Autodesk Inventor part; units mm, degrees
(part 2 of 8)
  line L645 (-14.4464, -63.849) -> (-14.5331, -63.849) construction
  spline S62 degree 2 poles (-14.5331, -63.849) (-14.5782, -63.849) (-14.6233, -63.8281) knots 0 0 0 1 1 1
  line L646 (-14.5331, -63.849) -> (-14.5782, -63.849) construction
  line L647 (-14.5782, -63.849) -> (-14.6233, -63.8281) construction
  spline S63 degree 2 poles (-14.6233, -63.8281) (-14.8315, -63.7379) (-14.9598, -63.5714) knots 0 0 0 1 1 1
  line L648 (-14.6233, -63.8281) -> (-14.8315, -63.7379) construction
  line L649 (-14.8315, -63.7379) -> (-14.9598, -63.5714) construction
  spline S64 degree 2 poles (-14.9598, -63.5714) (-15.2096, -63.8455) (-15.5774, -63.8455) knots 0 0 0 1 1 1
  line L650 (-14.9598, -63.5714) -> (-15.2096, -63.8455) construction
  line L651 (-15.2096, -63.8455) -> (-15.5774, -63.8455) construction
  spline S65 degree 2 poles (-4.8151, -52.1801) (-5.2315, -52.1801) (-5.2315, -51.7638) knots 0 0 0 1 1 1
  line L652 (-4.8151, -52.1801) -> (-5.2315, -52.1801) construction
  line L653 (-5.2315, -52.1801) -> (-5.2315, -51.7638) construction
  spline S66 degree 2 poles (-5.2315, -51.7638) (-5.2315, -51.3475) (-4.8151, -51.3475) knots 0 0 0 1 1 1
  line L654 (-5.2315, -51.7638) -> (-5.2315, -51.3475) construction
  line L655 (-5.2315, -51.3475) -> (-4.8151, -51.3475) construction
  line L656 (-4.8151, -51.3475) -> (-1.4915, -51.3475)
  spline S67 degree 2 poles (-1.4915, -51.3475) (-1.0821, -51.3475) (-1.0821, -51.7638) knots 0 0 0 1 1 1
  line L657 (-1.4915, -51.3475) -> (-1.0821, -51.3475) construction
  line L658 (-1.0821, -51.3475) -> (-1.0821, -51.7638) construction
  spline S68 degree 2 poles (-1.0821, -51.7638) (-1.0821, -52.1801) (-1.4915, -52.1801) knots 0 0 0 1 1 1
  line L659 (-1.0821, -51.7638) -> (-1.0821, -52.1801) construction
  line L660 (-1.0821, -52.1801) -> (-1.4915, -52.1801) construction
  line L661 (-1.4915, -52.1801) -> (-4.8151, -52.1801)
  spline S69 degree 2 poles (-9.8734, -55.9243) (-10.0004, -55.9243) (-10.0766, -55.8058) knots 0 0 0 1 1 1
  line L662 (-9.8734, -55.9243) -> (-10.0004, -55.9243) construction
  line L663 (-10.0004, -55.9243) -> (-10.0766, -55.8058) construction
  spline S70 degree 2 poles (-11.6765, -55.8058) (-11.7527, -55.9243) (-11.8797, -55.9243) knots 0 0 0 1 1 1
  line L664 (-11.6765, -55.8058) -> (-11.7527, -55.9243) construction
  line L665 (-11.7527, -55.9243) -> (-11.8797, -55.9243) construction
  spline S71 degree 2 poles (-11.8797, -55.9243) (-11.9812, -55.9243) (-12.1463, -55.7719) (-12.1463, -55.6661) knots 0 0 0 1 2 2 2
  line L666 (-11.8797, -55.9243) -> (-11.9812, -55.9243) construction
  line L667 (-11.9812, -55.9243) -> (-12.1463, -55.7719) construction
  line L668 (-12.1463, -55.7719) -> (-12.1463, -55.6661) construction
  spline S72 degree 2 poles (-12.1463, -55.6661) (-12.1463, -55.5942) (-12.104, -55.5222) knots 0 0 0 1 1 1
  line L669 (-12.1463, -55.6661) -> (-12.1463, -55.5942) construction
  line L670 (-12.1463, -55.5942) -> (-12.104, -55.5222) construction
  spline S73 degree 2 poles (-12.104, -52.771) (-12.1463, -52.6991) (-12.1463, -52.6271) knots 0 0 0 1 1 1
  line L671 (-12.104, -52.771) -> (-12.1463, -52.6991) construction
  line L672 (-12.1463, -52.6991) -> (-12.1463, -52.6271) construction
  spline S74 degree 2 poles (-12.1463, -52.6271) (-12.1463, -52.5213) (-11.9812, -52.3689) (-11.8797, -52.3689) knots 0 0 0 1 2 2 2
  line L673 (-12.1463, -52.6271) -> (-12.1463, -52.5213) construction
  line L674 (-12.1463, -52.5213) -> (-11.9812, -52.3689) construction
  line L675 (-11.9812, -52.3689) -> (-11.8797, -52.3689) construction
  spline S75 degree 2 poles (-11.8797, -52.3689) (-11.7527, -52.3689) (-11.6765, -52.4875) knots 0 0 0 1 1 1
  line L676 (-11.8797, -52.3689) -> (-11.7527, -52.3689) construction
  line L677 (-11.7527, -52.3689) -> (-11.6765, -52.4875) construction
  spline S76 degree 2 poles (-10.0766, -52.4875) (-10.0004, -52.3689) (-9.8734, -52.3689) knots 0 0 0 1 1 1
  line L678 (-10.0766, -52.4875) -> (-10.0004, -52.3689) construction
  line L679 (-10.0004, -52.3689) -> (-9.8734, -52.3689) construction
  spline S77 degree 2 poles (-9.8734, -52.3689) (-9.7718, -52.3689) (-9.6025, -52.5213) (-9.6025, -52.6271) knots 0 0 0 1 2 2 2
  line L680 (-9.8734, -52.3689) -> (-9.7718, -52.3689) construction
  line L681 (-9.7718, -52.3689) -> (-9.6025, -52.5213) construction
  line L682 (-9.6025, -52.5213) -> (-9.6025, -52.6271) construction
  spline S78 degree 2 poles (-9.6025, -52.6271) (-9.6025, -52.6991) (-9.6491, -52.771) knots 0 0 0 1 1 1
  line L683 (-9.6025, -52.6271) -> (-9.6025, -52.6991) construction
  line L684 (-9.6025, -52.6991) -> (-9.6491, -52.771) construction
  spline S79 degree 2 poles (-9.6491, -55.5222) (-9.6025, -55.5942) (-9.6025, -55.6661) knots 0 0 0 1 1 1
  line L685 (-9.6491, -55.5222) -> (-9.6025, -55.5942) construction
  line L686 (-9.6025, -55.5942) -> (-9.6025, -55.6661) construction
  spline S80 degree 2 poles (-9.6025, -55.6661) (-9.6025, -55.7719) (-9.7718, -55.9243) (-9.8734, -55.9243) knots 0 0 0 1 2 2 2
  line L687 (-9.6025, -55.6661) -> (-9.6025, -55.7719) construction
  line L688 (-9.6025, -55.7719) -> (-9.7718, -55.9243) construction
  line L689 (-9.7718, -55.9243) -> (-9.8734, -55.9243) construction
  spline S81 degree 2 poles (-18.3701, -55.6314) (-18.4645, -55.9145) (-18.6809, -55.9145) knots 0 0 0 1 1 1
  line L690 (-18.3701, -55.6314) -> (-18.4645, -55.9145) construction
  line L691 (-18.4645, -55.9145) -> (-18.6809, -55.9145) construction
  spline S82 degree 2 poles (-18.6809, -55.9145) (-18.903, -55.9145) (-18.9918, -55.6314) knots 0 0 0 1 1 1
  line L692 (-18.6809, -55.9145) -> (-18.903, -55.9145) construction
  line L693 (-18.903, -55.9145) -> (-18.9918, -55.6314) construction
  line L694 (-18.9918, -55.6314) -> (-20.9901, -49.7141)
  spline S83 degree 2 poles (-20.9901, -49.7141) (-21.0068, -49.6531) (-21.0068, -49.592) knots 0 0 0 1 1 1
  line L695 (-20.9901, -49.7141) -> (-21.0068, -49.6531) construction
  line L696 (-21.0068, -49.6531) -> (-21.0068, -49.592) construction
  spline S84 degree 2 poles (-21.0068, -49.592) (-21.0068, -49.2756) (-20.6626, -49.2756) knots 0 0 0 1 1 1
  line L697 (-21.0068, -49.592) -> (-21.0068, -49.2756) construction
  line L698 (-21.0068, -49.2756) -> (-20.6626, -49.2756) construction
  spline S85 degree 2 poles (-20.6626, -49.2756) (-20.4406, -49.2756) (-20.3629, -49.5032) knots 0 0 0 1 1 1
  line L699 (-20.6626, -49.2756) -> (-20.4406, -49.2756) construction
  line L700 (-20.4406, -49.2756) -> (-20.3629, -49.5032) construction
  spline S86 degree 2 poles (-16.999, -49.5032) (-16.9213, -49.2756) (-16.6993, -49.2756) knots 0 0 0 1 1 1
  line L701 (-16.999, -49.5032) -> (-16.9213, -49.2756) construction
  line L702 (-16.9213, -49.2756) -> (-16.6993, -49.2756) construction
  spline S87 degree 2 poles (-16.6993, -49.2756) (-16.3551, -49.2756) (-16.3551, -49.592) knots 0 0 0 1 1 1
  line L703 (-16.6993, -49.2756) -> (-16.3551, -49.2756) construction
  line L704 (-16.3551, -49.2756) -> (-16.3551, -49.592) construction
  spline S88 degree 2 poles (-16.3551, -49.592) (-16.3551, -49.6531) (-16.3773, -49.7141) knots 0 0 0 1 1 1
  line L705 (-16.3551, -49.592) -> (-16.3551, -49.6531) construction
  line L706 (-16.3551, -49.6531) -> (-16.3773, -49.7141) construction
  line L707 (-16.3773, -49.7141) -> (-18.3701, -55.6314)
  spline S89 degree 2 poles (14.3835, -40.7072) (14.1892, -40.7072) (13.9706, -40.95) (13.9706, -41.12) knots 0 0 0 1 2 2 2
  line L708 (14.3835, -40.7072) -> (14.1892, -40.7072) construction
  line L709 (14.1892, -40.7072) -> (13.9706, -40.95) construction
  line L710 (13.9706, -40.95) -> (13.9706, -41.12) construction
  spline S90 degree 2 poles (13.9706, -41.12) (13.9706, -41.29) (14.0747, -41.408) knots 0 0 0 1 1 1
  line L711 (13.9706, -41.12) -> (13.9706, -41.29) construction
  line L712 (13.9706, -41.29) -> (14.0747, -41.408) construction
  spline S91 degree 2 poles (14.0747, -41.408) (14.1892, -41.5364) (14.3835, -41.5364) knots 0 0 0 1 1 1
  line L713 (14.0747, -41.408) -> (14.1892, -41.5364) construction
  line L714 (14.1892, -41.5364) -> (14.3835, -41.5364) construction
  spline S92 degree 2 poles (13.9359, -43.1045) (13.8735, -43.2016) (13.7694, -43.2016) knots 0 0 0 1 1 1
  line L715 (13.9359, -43.1045) -> (13.8735, -43.2016) construction
  line L716 (13.8735, -43.2016) -> (13.7694, -43.2016) construction
  spline S93 degree 2 poles (13.7694, -43.2016) (13.6826, -43.2016) (13.5508, -43.0767) (13.5508, -42.9935) knots 0 0 0 1 2 2 2
  line L717 (13.7694, -43.2016) -> (13.6826, -43.2016) construction
  line L718 (13.6826, -43.2016) -> (13.5508, -43.0767) construction
  line L719 (13.5508, -43.0767) -> (13.5508, -42.9935) construction
  spline S94 degree 2 poles (13.5508, -42.9935) (13.5508, -42.931) (13.589, -42.8755) knots 0 0 0 1 1 1
  line L720 (13.5508, -42.9935) -> (13.5508, -42.931) construction
  line L721 (13.5508, -42.931) -> (13.589, -42.8755) construction
  line L722 (13.589, -42.8755) -> (14.2135, -41.9388)
  spline S95 degree 2 poles (14.2135, -41.9388) (13.9012, -41.8868) (13.7173, -41.6404) knots 0 0 0 1 1 1
  line L723 (14.2135, -41.9388) -> (13.9012, -41.8868) construction
  line L724 (13.9012, -41.8868) -> (13.7173, -41.6404) construction
  spline S96 degree 2 poles (13.7173, -41.6404) (13.5543, -41.4184) (13.5543, -41.12) knots 0 0 0 1 1 1
  line L725 (13.7173, -41.6404) -> (13.5543, -41.4184) construction
  line L726 (13.5543, -41.4184) -> (13.5543, -41.12) construction
  spline S97 degree 2 poles (13.5543, -41.12) (13.5543, -40.7835) (13.7624, -40.5511) knots 0 0 0 1 1 1
  line L727 (13.5543, -41.12) -> (13.5543, -40.7835) construction
  line L728 (13.5543, -40.7835) -> (13.7624, -40.5511) construction
  spline S98 degree 2 poles (13.7624, -40.5511) (13.9914, -40.2909) (14.3835, -40.2909) knots 0 0 0 1 1 1
  line L729 (13.7624, -40.5511) -> (13.9914, -40.2909) construction
  line L730 (13.9914, -40.2909) -> (14.3835, -40.2909) construction
  line L731 (14.3835, -40.2909) -> (15.4208, -40.2909)
  spline S99 degree 2 poles (15.4208, -40.2909) (15.6289, -40.2909) (15.6289, -40.499) knots 0 0 0 1 1 1
  line L732 (15.4208, -40.2909) -> (15.6289, -40.2909) construction
  line L733 (15.6289, -40.2909) -> (15.6289, -40.499) construction
  line L734 (15.6289, -40.499) -> (15.6289, -42.99)
  spline S100 degree 2 poles (15.6289, -42.99) (15.6289, -43.1982) (15.4208, -43.1982) knots 0 0 0 1 1 1
  line L735 (15.6289, -42.99) -> (15.6289, -43.1982) construction
  line L736 (15.6289, -43.1982) -> (15.4208, -43.1982) construction
  spline S101 degree 2 poles (15.4208, -43.1982) (15.2126, -43.1982) (15.2126, -42.99) knots 0 0 0 1 1 1
  line L737 (15.4208, -43.1982) -> (15.2126, -43.1982) construction
  line L738 (15.2126, -43.1982) -> (15.2126, -42.99) construction
  spline S102 degree 2 poles (11.8925, -42.7819) (12.0625, -42.7819) (12.3053, -42.5355) (12.3053, -42.3655) knots 0 0 0 1 2 2 2
  line L739 (11.8925, -42.7819) -> (12.0625, -42.7819) construction
  line L740 (12.0625, -42.7819) -> (12.3053, -42.5355) construction
  line L741 (12.3053, -42.5355) -> (12.3053, -42.3655) construction
  spline S103 degree 2 poles (11.4762, -40.7072) (11.3062, -40.7072) (11.0633, -40.9535) (11.0633, -41.1235) knots 0 0 0 1 2 2 2
  line L742 (11.4762, -40.7072) -> (11.3062, -40.7072) construction
  line L743 (11.3062, -40.7072) -> (11.0633, -40.9535) construction
  line L744 (11.0633, -40.9535) -> (11.0633, -41.1235) construction
  line L745 (11.0633, -41.1235) -> (11.0633, -42.3655)
  spline S104 degree 2 poles (11.0633, -42.3655) (11.0633, -42.5355) (11.3062, -42.7819) (11.4762, -42.7819) knots 0 0 0 1 2 2 2
  line L746 (11.0633, -42.3655) -> (11.0633, -42.5355) construction
  line L747 (11.0633, -42.5355) -> (11.3062, -42.7819) construction
  line L748 (11.3062, -42.7819) -> (11.4762, -42.7819) construction
  line L749 (11.4762, -42.7819) -> (11.8925, -42.7819)
  line L750 (11.8925, -43.1982) -> (11.4762, -43.1982)
  spline S105 degree 2 poles (11.4762, -43.1982) (11.1362, -43.1982) (10.647, -42.7125) (10.647, -42.369) knots 0 0 0 1 2 2 2
  line L751 (11.4762, -43.1982) -> (11.1362, -43.1982) construction
  line L752 (11.1362, -43.1982) -> (10.647, -42.7125) construction
  line L753 (10.647, -42.7125) -> (10.647, -42.369) construction
  line L754 (10.647, -42.369) -> (10.647, -41.12)
  spline S106 degree 2 poles (10.647, -41.12) (10.647, -40.7766) (11.1362, -40.2909) (11.4762, -40.2909) knots 0 0 0 1 2 2 2
  line L755 (10.647, -41.12) -> (10.647, -40.7766) construction
  line L756 (10.647, -40.7766) -> (11.1362, -40.2909) construction
  line L757 (11.1362, -40.2909) -> (11.4762, -40.2909) construction
  line L758 (11.4762, -40.2909) -> (12.5135, -40.2909)
  spline S107 degree 2 poles (12.5135, -40.2909) (12.7216, -40.2909) (12.7216, -40.499) knots 0 0 0 1 1 1
  line L759 (12.5135, -40.2909) -> (12.7216, -40.2909) construction
  line L760 (12.7216, -40.2909) -> (12.7216, -40.499) construction
  line L761 (12.7216, -40.499) -> (12.7216, -42.3621)
  spline S108 degree 2 poles (12.7216, -42.3621) (12.7216, -42.6743) (13.0131, -42.7992) knots 0 0 0 1 1 1
  line L762 (12.7216, -42.3621) -> (12.7216, -42.6743) construction
  line L763 (12.7216, -42.6743) -> (13.0131, -42.7992) construction
  spline S109 degree 2 poles (13.0131, -42.7992) (13.1414, -42.8512) (13.1414, -42.9831) knots 0 0 0 1 1 1
  line L764 (13.0131, -42.7992) -> (13.1414, -42.8512) construction
  line L765 (13.1414, -42.8512) -> (13.1414, -42.9831) construction
  spline S110 degree 2 poles (13.1414, -42.9831) (13.1414, -43.0698) (13.0235, -43.2016) (12.9367, -43.2016) knots 0 0 0 1 2 2 2
  line L766 (13.1414, -42.9831) -> (13.1414, -43.0698) construction
  line L767 (13.1414, -43.0698) -> (13.0235, -43.2016) construction
  line L768 (13.0235, -43.2016) -> (12.9367, -43.2016) construction
  spline S111 degree 2 poles (12.9367, -43.2016) (12.8916, -43.2016) (12.8465, -43.1808) knots 0 0 0 1 1 1
  line L769 (12.9367, -43.2016) -> (12.8916, -43.2016) construction
  line L770 (12.8916, -43.2016) -> (12.8465, -43.1808) construction
  spline S112 degree 2 poles (12.8465, -43.1808) (12.6384, -43.0906) (12.51, -42.9241) knots 0 0 0 1 1 1
  line L771 (12.8465, -43.1808) -> (12.6384, -43.0906) construction
  line L772 (12.6384, -43.0906) -> (12.51, -42.9241) construction
  spline S113 degree 2 poles (12.51, -42.9241) (12.2602, -43.1982) (11.8925, -43.1982) knots 0 0 0 1 1 1
  line L773 (12.51, -42.9241) -> (12.2602, -43.1982) construction
  line L774 (12.2602, -43.1982) -> (11.8925, -43.1982) construction
  spline S114 degree 2 poles (-0.7775, -43.1982) (-0.9857, -43.1982) (-0.9857, -42.99) knots 0 0 0 1 1 1
  line L775 (-0.7775, -43.1982) -> (-0.9857, -43.1982) construction
  line L776 (-0.9857, -43.1982) -> (-0.9857, -42.99) construction
  spline S115 degree 2 poles (-2.2416, -43.0559) (-2.2867, -43.1982) (-2.4255, -43.1982) knots 0 0 0 1 1 1
  line L777 (-2.2416, -43.0559) -> (-2.2867, -43.1982) construction
  line L778 (-2.2867, -43.1982) -> (-2.4255, -43.1982) construction
  spline S116 degree 2 poles (-2.4255, -43.1982) (-2.644, -43.1982) (-2.644, -43.0004) knots 0 0 0 1 1 1
  line L779 (-2.4255, -43.1982) -> (-2.644, -43.1982) construction
  line L780 (-2.644, -43.1982) -> (-2.644, -43.0004) construction
  spline S117 degree 2 poles (-2.644, -43.0004) (-2.644, -42.9623) (-2.6301, -42.9241) knots 0 0 0 1 1 1
  line L781 (-2.644, -43.0004) -> (-2.644, -42.9623) construction
  line L782 (-2.644, -42.9623) -> (-2.6301, -42.9241) construction
  line L783 (-2.6301, -42.9241) -> (-1.8079, -40.4331)
  spline S118 degree 2 poles (-1.8079, -40.4331) (-1.7628, -40.2909) (-1.6136, -40.2909) knots 0 0 0 1 1 1
  line L784 (-1.8079, -40.4331) -> (-1.7628, -40.2909) construction
  line L785 (-1.7628, -40.2909) -> (-1.6136, -40.2909) construction
  line L786 (-1.6136, -40.2909) -> (-0.7775, -40.2909)
  spline S119 degree 2 poles (-0.7775, -40.2909) (-0.5694, -40.2909) (-0.5694, -40.499) knots 0 0 0 1 1 1
  line L787 (-0.7775, -40.2909) -> (-0.5694, -40.2909) construction
  line L788 (-0.5694, -40.2909) -> (-0.5694, -40.499) construction
  line L789 (-0.5694, -40.499) -> (-0.5694, -42.99)
  spline S120 degree 2 poles (-0.5694, -42.99) (-0.5694, -43.1982) (-0.7775, -43.1982) knots 0 0 0 1 1 1
  line L790 (-0.5694, -42.99) -> (-0.5694, -43.1982) construction
  line L791 (-0.5694, -43.1982) -> (-0.7775, -43.1982) construction
  spline S121 degree 2 poles (-12.4067, -43.1982) (-12.6149, -43.1982) (-12.6149, -42.99) knots 0 0 0 1 1 1
  line L792 (-12.4067, -43.1982) -> (-12.6149, -43.1982) construction
  line L793 (-12.6149, -43.1982) -> (-12.6149, -42.99) construction
  line L794 (-12.6149, -42.99) -> (-12.6149, -41.1235)
  spline S122 degree 2 poles (-12.6149, -41.1235) (-12.6149, -40.9535) (-12.8577, -40.7072) (-13.0277, -40.7072) knots 0 0 0 1 2 2 2
  line L795 (-12.6149, -41.1235) -> (-12.6149, -40.9535) construction
  line L796 (-12.6149, -40.9535) -> (-12.8577, -40.7072) construction
  line L797 (-12.8577, -40.7072) -> (-13.0277, -40.7072) construction
  spline S123 degree 2 poles (-13.8569, -42.99) (-13.8569, -43.1982) (-14.0651, -43.1982) knots 0 0 0 1 1 1
  line L798 (-13.8569, -42.99) -> (-13.8569, -43.1982) construction
  line L799 (-13.8569, -43.1982) -> (-14.0651, -43.1982) construction
  spline S124 degree 2 poles (-14.0651, -43.1982) (-14.2732, -43.1982) (-14.2732, -42.99) knots 0 0 0 1 1 1
  line L800 (-14.0651, -43.1982) -> (-14.2732, -43.1982) construction
  line L801 (-14.2732, -43.1982) -> (-14.2732, -42.99) construction
  line L802 (-14.2732, -42.99) -> (-14.2732, -40.499)
  spline S125 degree 2 poles (-14.2732, -40.499) (-14.2732, -40.2909) (-14.0651, -40.2909) knots 0 0 0 1 1 1
  line L803 (-14.2732, -40.499) -> (-14.2732, -40.2909) construction
  line L804 (-14.2732, -40.2909) -> (-14.0651, -40.2909) construction
  line L805 (-14.0651, -40.2909) -> (-13.0277, -40.2909)
  spline S126 degree 2 poles (-13.0277, -40.2909) (-12.6843, -40.2909) (-12.1986, -40.7766) (-12.1986, -41.12) knots 0 0 0 1 2 2 2
  line L806 (-13.0277, -40.2909) -> (-12.6843, -40.2909) construction
  line L807 (-12.6843, -40.2909) -> (-12.1986, -40.7766) construction
  line L808 (-12.1986, -40.7766) -> (-12.1986, -41.12) construction
  line L809 (-12.1986, -41.12) -> (-12.1986, -42.99)
  spline S127 degree 2 poles (-12.1986, -42.99) (-12.1986, -43.1982) (-12.4067, -43.1982) knots 0 0 0 1 1 1
  line L810 (-12.1986, -42.99) -> (-12.1986, -43.1982) construction
  line L811 (-12.1986, -43.1982) -> (-12.4067, -43.1982) construction
  spline S128 degree 2 poles (-15.935, -42.7819) (-15.765, -42.7819) (-15.5222, -42.5355) (-15.5222, -42.3655) knots 0 0 0 1 2 2 2
  line L812 (-15.935, -42.7819) -> (-15.765, -42.7819) construction
  line L813 (-15.765, -42.7819) -> (-15.5222, -42.5355) construction
  line L814 (-15.5222, -42.5355) -> (-15.5222, -42.3655) construction
  spline S129 degree 2 poles (-16.3514, -40.7072) (-16.5213, -40.7072) (-16.7642, -40.9535) (-16.7642, -41.1235) knots 0 0 0 1 2 2 2
  line L815 (-16.3514, -40.7072) -> (-16.5213, -40.7072) construction
  line L816 (-16.5213, -40.7072) -> (-16.7642, -40.9535) construction
  line L817 (-16.7642, -40.9535) -> (-16.7642, -41.1235) construction
  line L818 (-16.7642, -41.1235) -> (-16.7642, -42.3655)
  spline S130 degree 2 poles (-16.7642, -42.3655) (-16.7642, -42.5355) (-16.5213, -42.7819) (-16.3514, -42.7819) knots 0 0 0 1 2 2 2
  line L819 (-16.7642, -42.3655) -> (-16.7642, -42.5355) construction
  line L820 (-16.7642, -42.5355) -> (-16.5213, -42.7819) construction
  line L821 (-16.5213, -42.7819) -> (-16.3514, -42.7819) construction
  line L822 (-16.3514, -42.7819) -> (-15.935, -42.7819)
  line L823 (-15.935, -43.1982) -> (-16.3514, -43.1982)
  spline S131 degree 2 poles (-16.3514, -43.1982) (-16.6913, -43.1982) (-17.1805, -42.7125) (-17.1805, -42.369) knots 0 0 0 1 2 2 2
  line L824 (-16.3514, -43.1982) -> (-16.6913, -43.1982) construction
  line L825 (-16.6913, -43.1982) -> (-17.1805, -42.7125) construction
  line L826 (-17.1805, -42.7125) -> (-17.1805, -42.369) construction
  line L827 (-17.1805, -42.369) -> (-17.1805, -41.12)
  spline S132 degree 2 poles (-17.1805, -41.12) (-17.1805, -40.7766) (-16.6913, -40.2909) (-16.3514, -40.2909) knots 0 0 0 1 2 2 2
  line L828 (-17.1805, -41.12) -> (-17.1805, -40.7766) construction
  line L829 (-17.1805, -40.7766) -> (-16.6913, -40.2909) construction
  line L830 (-16.6913, -40.2909) -> (-16.3514, -40.2909) construction
  line L831 (-16.3514, -40.2909) -> (-15.314, -40.2909)
  spline S133 degree 2 poles (-15.314, -40.2909) (-15.1059, -40.2909) (-15.1059, -40.499) knots 0 0 0 1 1 1
  line L832 (-15.314, -40.2909) -> (-15.1059, -40.2909) construction
  line L833 (-15.1059, -40.2909) -> (-15.1059, -40.499) construction
  line L834 (-15.1059, -40.499) -> (-15.1059, -42.3621)
  spline S134 degree 2 poles (-15.1059, -42.3621) (-15.1059, -42.6743) (-14.8144, -42.7992) knots 0 0 0 1 1 1
  line L835 (-15.1059, -42.3621) -> (-15.1059, -42.6743) construction
  line L836 (-15.1059, -42.6743) -> (-14.8144, -42.7992) construction
  spline S135 degree 2 poles (-14.8144, -42.7992) (-14.6861, -42.8512) (-14.6861, -42.9831) knots 0 0 0 1 1 1
  line L837 (-14.8144, -42.7992) -> (-14.6861, -42.8512) construction
  line L838 (-14.6861, -42.8512) -> (-14.6861, -42.9831) construction
  spline S136 degree 2 poles (-14.6861, -42.9831) (-14.6861, -43.0698) (-14.804, -43.2016) (-14.8908, -43.2016) knots 0 0 0 1 2 2 2
  line L839 (-14.6861, -42.9831) -> (-14.6861, -43.0698) construction
  line L840 (-14.6861, -43.0698) -> (-14.804, -43.2016) construction
  line L841 (-14.804, -43.2016) -> (-14.8908, -43.2016) construction
  spline S137 degree 2 poles (-14.8908, -43.2016) (-14.9359, -43.2016) (-14.981, -43.1808) knots 0 0 0 1 1 1
  line L842 (-14.8908, -43.2016) -> (-14.9359, -43.2016) construction
  line L843 (-14.9359, -43.2016) -> (-14.981, -43.1808) construction
  spline S138 degree 2 poles (-14.981, -43.1808) (-15.1891, -43.0906) (-15.3175, -42.9241) knots 0 0 0 1 1 1
  line L844 (-14.981, -43.1808) -> (-15.1891, -43.0906) construction
  line L845 (-15.1891, -43.0906) -> (-15.3175, -42.9241) construction
  spline S139 degree 2 poles (-15.3175, -42.9241) (-15.5673, -43.1982) (-15.935, -43.1982) knots 0 0 0 1 1 1
  line L846 (-15.3175, -42.9241) -> (-15.5673, -43.1982) construction
  line L847 (-15.5673, -43.1982) -> (-15.935, -43.1982) construction
  spline S140 degree 2 poles (12.063, -33.4278) (11.723, -33.4278) (11.2304, -32.9421) (11.2304, -32.5987) knots 0 0 0 1 2 2 2
  line L848 (12.063, -33.4278) -> (11.723, -33.4278) construction
  line L849 (11.723, -33.4278) -> (11.2304, -32.9421) construction
  line L850 (11.2304, -32.9421) -> (11.2304, -32.5987) construction
  line L851 (11.2304, -32.5987) -> (11.2304, -31.3497)
  spline S141 degree 2 poles (11.2304, -31.3497) (11.2304, -31.0062) (11.723, -30.5205) (12.063, -30.5205) knots 0 0 0 1 2 2 2
  line L852 (11.2304, -31.3497) -> (11.2304, -31.0062) construction
  line L853 (11.2304, -31.0062) -> (11.723, -30.5205) construction
  line L854 (11.723, -30.5205) -> (12.063, -30.5205) construction
  line L855 (12.063, -30.5205) -> (12.684, -30.5205)
  spline S142 degree 2 poles (12.684, -30.5205) (12.8922, -30.5205) (12.8922, -30.7287) knots 0 0 0 1 1 1
  line L856 (12.684, -30.5205) -> (12.8922, -30.5205) construction
  line L857 (12.8922, -30.5205) -> (12.8922, -30.7287) construction
  spline S143 degree 2 poles (12.8922, -30.7287) (12.8922, -30.9369) (12.684, -30.9369) knots 0 0 0 1 1 1
  line L858 (12.8922, -30.7287) -> (12.8922, -30.9369) construction
  line L859 (12.8922, -30.9369) -> (12.684, -30.9369) construction
  line L860 (12.684, -30.9369) -> (12.063, -30.9369)
  spline S144 degree 2 poles (12.063, -30.9369) (11.893, -30.9369) (11.6467, -31.1832) (11.6467, -31.3532) knots 0 0 0 1 2 2 2
  line L861 (12.063, -30.9369) -> (11.893, -30.9369) construction
  line L862 (11.893, -30.9369) -> (11.6467, -31.1832) construction
  line L863 (11.6467, -31.1832) -> (11.6467, -31.3532) construction
  line L864 (11.6467, -31.3532) -> (11.6467, -32.5952)
  spline S145 degree 2 poles (11.6467, -32.5952) (11.6467, -32.7652) (11.893, -33.0115) (12.063, -33.0115) knots 0 0 0 1 2 2 2
  line L865 (11.6467, -32.5952) -> (11.6467, -32.7652) construction
  line L866 (11.6467, -32.7652) -> (11.893, -33.0115) construction
  line L867 (11.893, -33.0115) -> (12.063, -33.0115) construction
  line L868 (12.063, -33.0115) -> (12.684, -33.0115)
  spline S146 degree 2 poles (12.684, -33.0115) (12.8922, -33.0115) (12.8922, -33.2197) knots 0 0 0 1 1 1
  line L869 (12.684, -33.0115) -> (12.8922, -33.0115) construction
  line L870 (12.8922, -33.0115) -> (12.8922, -33.2197) construction
  spline S147 degree 2 poles (12.8922, -33.2197) (12.8922, -33.4278) (12.684, -33.4278) knots 0 0 0 1 1 1
  line L871 (12.8922, -33.2197) -> (12.8922, -33.4278) construction
  line L872 (12.8922, -33.4278) -> (12.684, -33.4278) construction
  line L873 (12.684, -33.4278) -> (12.063, -33.4278)
  spline S148 degree 2 poles (22.4086, -21.7323) (22.6167, -21.7323) (22.6167, -21.9405) knots 0 0 0 1 1 1
  line L874 (22.4086, -21.7323) -> (22.6167, -21.7323) construction
  line L875 (22.6167, -21.7323) -> (22.6167, -21.9405) construction
  spline S149 degree 2 poles (22.6167, -21.9405) (22.6167, -22.1486) (22.4086, -22.1486) knots 0 0 0 1 1 1
  line L876 (22.6167, -21.9405) -> (22.6167, -22.1486) construction
  line L877 (22.6167, -22.1486) -> (22.4086, -22.1486) construction
  spline S150 degree 2 poles (22.4086, -22.1486) (22.2004, -22.1486) (22.2004, -21.9405) knots 0 0 0 1 1 1
  line L878 (22.4086, -22.1486) -> (22.2004, -22.1486) construction
  line L879 (22.2004, -22.1486) -> (22.2004, -21.9405) construction
  spline S151 degree 2 poles (22.2004, -21.9405) (22.2004, -21.7323) (22.4086, -21.7323) knots 0 0 0 1 1 1
  line L880 (22.2004, -21.9405) -> (22.2004, -21.7323) construction
  line L881 (22.2004, -21.7323) -> (22.4086, -21.7323) construction
  spline S152 degree 2 poles (20.5386, -21.7323) (20.7086, -21.7323) (20.9515, -21.486) (20.9515, -21.316) knots 0 0 0 1 2 2 2
  line L882 (20.5386, -21.7323) -> (20.7086, -21.7323) construction
  line L883 (20.7086, -21.7323) -> (20.9515, -21.486) construction
  line L884 (20.9515, -21.486) -> (20.9515, -21.316) construction
  line L885 (20.9515, -21.316) -> (20.9515, -20.074)
  spline S153 degree 2 poles (20.9515, -20.074) (20.9515, -19.904) (20.7086, -19.6576) (20.5386, -19.6576) knots 0 0 0 1 2 2 2
  line L886 (20.9515, -20.074) -> (20.9515, -19.904) construction
  line L887 (20.9515, -19.904) -> (20.7086, -19.6576) construction
  line L888 (20.7086, -19.6576) -> (20.5386, -19.6576) construction
  spline S154 degree 2 poles (19.7094, -23.186) (19.7094, -23.3941) (19.5013, -23.3941) knots 0 0 0 1 1 1
  line L889 (19.7094, -23.186) -> (19.7094, -23.3941) construction
  line L890 (19.7094, -23.3941) -> (19.5013, -23.3941) construction
  spline S155 degree 2 poles (19.5013, -23.3941) (19.2931, -23.3941) (19.2931, -23.186) knots 0 0 0 1 1 1
  line L891 (19.5013, -23.3941) -> (19.2931, -23.3941) construction
  line L892 (19.2931, -23.3941) -> (19.2931, -23.186) construction
  line L893 (19.2931, -23.186) -> (19.2931, -19.4495)
  spline S156 degree 2 poles (19.2931, -19.4495) (19.2931, -19.2413) (19.5013, -19.2413) knots 0 0 0 1 1 1
  line L894 (19.2931, -19.4495) -> (19.2931, -19.2413) construction
  line L895 (19.2931, -19.2413) -> (19.5013, -19.2413) construction
  line L896 (19.5013, -19.2413) -> (20.5386, -19.2413)
  spline S157 degree 2 poles (20.5386, -19.2413) (20.8821, -19.2413) (21.3678, -19.727) (21.3678, -20.0705) knots 0 0 0 1 2 2 2
  line L897 (20.5386, -19.2413) -> (20.8821, -19.2413) construction
  line L898 (20.8821, -19.2413) -> (21.3678, -19.727) construction
  line L899 (21.3678, -19.727) -> (21.3678, -20.0705) construction
  line L900 (21.3678, -20.0705) -> (21.3678, -21.3195)
  spline S158 degree 2 poles (21.3678, -21.3195) (21.3678, -21.6629) (20.8821, -22.1486) (20.5386, -22.1486) knots 0 0 0 1 2 2 2
  line L901 (21.3678, -21.3195) -> (21.3678, -21.6629) construction
  line L902 (21.3678, -21.6629) -> (20.8821, -22.1486) construction
  line L903 (20.8821, -22.1486) -> (20.5386, -22.1486) construction
  spline S159 degree 2 poles (18.0442, -20.0705) (18.0442, -19.9005) (17.8013, -19.6576) (17.6313, -19.6576) knots 0 0 0 1 2 2 2
  line L904 (18.0442, -20.0705) -> (18.0442, -19.9005) construction
  line L905 (18.0442, -19.9005) -> (17.8013, -19.6576) construction
  line L906 (17.8013, -19.6576) -> (17.6313, -19.6576) construction
  line L907 (17.6313, -19.6576) -> (17.215, -19.6576)
  spline S160 degree 2 poles (17.215, -19.6576) (17.045, -19.6576) (16.8021, -19.9005) (16.8021, -20.0705) knots 0 0 0 1 2 2 2
  line L908 (17.215, -19.6576) -> (17.045, -19.6576) construction
  line L909 (17.045, -19.6576) -> (16.8021, -19.9005) construction
  line L910 (16.8021, -19.9005) -> (16.8021, -20.0705) construction
  spline S161 degree 2 poles (16.8021, -21.316) (16.8021, -21.486) (17.0485, -21.7323) (17.2185, -21.7323) knots 0 0 0 1 2 2 2
  line L911 (16.8021, -21.316) -> (16.8021, -21.486) construction
  line L912 (16.8021, -21.486) -> (17.0485, -21.7323) construction
  line L913 (17.0485, -21.7323) -> (17.2185, -21.7323) construction
  line L914 (17.2185, -21.7323) -> (18.2523, -21.7323)
  spline S162 degree 2 poles (18.2523, -21.7323) (18.4605, -21.7323) (18.4605, -21.9405) knots 0 0 0 1 1 1
  line L915 (18.2523, -21.7323) -> (18.4605, -21.7323) construction
  line L916 (18.4605, -21.7323) -> (18.4605, -21.9405) construction
  spline S163 degree 2 poles (18.4605, -21.9405) (18.4605, -22.1486) (18.2523, -22.1486) knots 0 0 0 1 1 1
  line L917 (18.4605, -21.9405) -> (18.4605, -22.1486) construction
  line L918 (18.4605, -22.1486) -> (18.2523, -22.1486) construction
  line L919 (18.2523, -22.1486) -> (17.215, -22.1486)
  spline S164 degree 2 poles (17.215, -22.1486) (16.8715, -22.1486) (16.3858, -21.6629) (16.3858, -21.3195) knots 0 0 0 1 2 2 2
  line L920 (17.215, -22.1486) -> (16.8715, -22.1486) construction
  line L921 (16.8715, -22.1486) -> (16.3858, -21.6629) construction
  line L922 (16.3858, -21.6629) -> (16.3858, -21.3195) construction
  line L923 (16.3858, -21.3195) -> (16.3858, -20.0705)
  spline S165 degree 2 poles (16.3858, -20.0705) (16.3858, -19.727) (16.8715, -19.2413) (17.215, -19.2413) knots 0 0 0 1 2 2 2
  line L924 (16.3858, -20.0705) -> (16.3858, -19.727) construction
  line L925 (16.3858, -19.727) -> (16.8715, -19.2413) construction
  line L926 (16.8715, -19.2413) -> (17.215, -19.2413) construction
  line L927 (17.215, -19.2413) -> (17.6313, -19.2413)
  spline S166 degree 2 poles (17.6313, -19.2413) (17.9748, -19.2413) (18.4605, -19.727) (18.4605, -20.0705) knots 0 0 0 1 2 2 2
  line L928 (17.6313, -19.2413) -> (17.9748, -19.2413) construction
  line L929 (17.9748, -19.2413) -> (18.4605, -19.727) construction
  line L930 (18.4605, -19.727) -> (18.4605, -20.0705) construction
  line L931 (18.4605, -20.0705) -> (18.4605, -20.695)
  spline S167 degree 2 poles (18.4605, -20.695) (18.4605, -20.9031) (18.2523, -20.9031) knots 0 0 0 1 1 1
  line L932 (18.4605, -20.695) -> (18.4605, -20.9031) construction
  line L933 (18.4605, -20.9031) -> (18.2523, -20.9031) construction
  spline S168 degree 2 poles (11.1922, -20.9031) (10.9841, -20.9031) (10.9841, -20.695) knots 0 0 0 1 1 1
  line L934 (11.1922, -20.9031) -> (10.9841, -20.9031) construction
  line L935 (10.9841, -20.9031) -> (10.9841, -20.695) construction
  spline S169 degree 2 poles (10.9841, -20.695) (10.9841, -20.4868) (11.1922, -20.4868) knots 0 0 0 1 1 1
  line L936 (10.9841, -20.695) -> (10.9841, -20.4868) construction
  line L937 (10.9841, -20.4868) -> (11.1922, -20.4868) construction
  line L938 (11.1922, -20.4868) -> (11.4004, -20.4868)
  spline S170 degree 2 poles (11.4004, -20.4868) (11.5947, -20.4868) (11.7092, -20.3585) knots 0 0 0 1 1 1
  line L939 (11.4004, -20.4868) -> (11.5947, -20.4868) construction
  line L940 (11.5947, -20.4868) -> (11.7092, -20.3585) construction
  spline S171 degree 2 poles (11.7092, -20.3585) (11.8132, -20.2405) (11.8132, -20.0705) knots 0 0 0 1 1 1
  line L941 (11.7092, -20.3585) -> (11.8132, -20.2405) construction
  line L942 (11.8132, -20.2405) -> (11.8132, -20.0705) construction
  spline S172 degree 2 poles (11.8132, -20.0705) (11.8132, -19.9005) (11.7092, -19.786) knots 0 0 0 1 1 1
  line L943 (11.8132, -20.0705) -> (11.8132, -19.9005) construction
  line L944 (11.8132, -19.9005) -> (11.7092, -19.786) construction
  spline S173 degree 2 poles (11.7092, -19.786) (11.5947, -19.6576) (11.3969, -19.6576) knots 0 0 0 1 1 1
  line L945 (11.7092, -19.786) -> (11.5947, -19.6576) construction
  line L946 (11.5947, -19.6576) -> (11.3969, -19.6576) construction
  line L947 (11.3969, -19.6576) -> (11.1888, -19.6576)
  spline S174 degree 2 poles (11.1888, -19.6576) (10.9078, -19.6576) (10.6927, -19.8242) knots 0 0 0 1 1 1
  line L948 (11.1888, -19.6576) -> (10.9078, -19.6576) construction
  line L949 (10.9078, -19.6576) -> (10.6927, -19.8242) construction
  spline S175 degree 2 poles (10.6927, -19.8242) (10.6302, -19.8693) (10.5643, -19.8693) knots 0 0 0 1 1 1
  line L950 (10.6927, -19.8242) -> (10.6302, -19.8693) construction
  line L951 (10.6302, -19.8693) -> (10.5643, -19.8693) construction
  spline S176 degree 2 poles (10.5643, -19.8693) (10.481, -19.8693) (10.3561, -19.7409) (10.3561, -19.6542) knots 0 0 0 1 2 2 2
  line L952 (10.5643, -19.8693) -> (10.481, -19.8693) construction
  line L953 (10.481, -19.8693) -> (10.3561, -19.7409) construction
  line L954 (10.3561, -19.7409) -> (10.3561, -19.6542) construction
  spline S177 degree 2 poles (10.3561, -19.6542) (10.3561, -19.557) (10.4429, -19.4911) knots 0 0 0 1 1 1
  line L955 (10.3561, -19.6542) -> (10.3561, -19.557) construction
  line L956 (10.3561, -19.557) -> (10.4429, -19.4911) construction
  spline S178 degree 2 poles (10.4429, -19.4911) (10.7655, -19.2413) (11.1888, -19.2413) knots 0 0 0 1 1 1
  line L957 (10.4429, -19.4911) -> (10.7655, -19.2413) construction
  line L958 (10.7655, -19.2413) -> (11.1888, -19.2413) construction
  line L959 (11.1888, -19.2413) -> (11.3969, -19.2413)
  spline S179 degree 2 poles (11.3969, -19.2413) (11.789, -19.2413) (12.0214, -19.4981) knots 0 0 0 1 1 1
  line L960 (11.3969, -19.2413) -> (11.789, -19.2413) construction
  line L961 (11.789, -19.2413) -> (12.0214, -19.4981) construction
  spline S180 degree 2 poles (12.0214, -19.4981) (12.2296, -19.734) (12.2296, -20.0705) knots 0 0 0 1 1 1
  line L962 (12.0214, -19.4981) -> (12.2296, -19.734) construction
  line L963 (12.2296, -19.734) -> (12.2296, -20.0705) construction
  spline S181 degree 2 poles (12.2296, -20.0705) (12.2296, -20.4556) (11.9694, -20.695) knots 0 0 0 1 1 1
  line L964 (12.2296, -20.0705) -> (12.2296, -20.4556) construction
  line L965 (12.2296, -20.4556) -> (11.9694, -20.695) construction
  spline S182 degree 2 poles (11.9694, -20.695) (12.2296, -20.9344) (12.2296, -21.3195) knots 0 0 0 1 1 1
  line L966 (11.9694, -20.695) -> (12.2296, -20.9344) construction
  line L967 (12.2296, -20.9344) -> (12.2296, -21.3195) construction
  spline S183 degree 2 poles (12.2296, -21.3195) (12.2296, -21.6594) (12.0214, -21.8919) knots 0 0 0 1 1 1
  line L968 (12.2296, -21.3195) -> (12.2296, -21.6594) construction
  line L969 (12.2296, -21.6594) -> (12.0214, -21.8919) construction
  spline S184 degree 2 poles (12.0214, -21.8919) (11.789, -22.1486) (11.3969, -22.1486) knots 0 0 0 1 1 1
  line L970 (12.0214, -21.8919) -> (11.789, -22.1486) construction
  line L971 (11.789, -22.1486) -> (11.3969, -22.1486) construction
  line L972 (11.3969, -22.1486) -> (11.1888, -22.1486)
  spline S185 degree 2 poles (11.1888, -22.1486) (10.7655, -22.1486) (10.4429, -21.8988) knots 0 0 0 1 1 1
  line L973 (11.1888, -22.1486) -> (10.7655, -22.1486) construction
  line L974 (10.7655, -22.1486) -> (10.4429, -21.8988) construction
  spline S186 degree 2 poles (10.4429, -21.8988) (10.3561, -21.8329) (10.3561, -21.7358) knots 0 0 0 1 1 1
  line L975 (10.4429, -21.8988) -> (10.3561, -21.8329) construction
  line L976 (10.3561, -21.8329) -> (10.3561, -21.7358) construction
  spline S187 degree 2 poles (10.3561, -21.7358) (10.3561, -21.649) (10.481, -21.5207) (10.5643, -21.5207) knots 0 0 0 1 2 2 2
  line L977 (10.3561, -21.7358) -> (10.3561, -21.649) construction
  line L978 (10.3561, -21.649) -> (10.481, -21.5207) construction
  line L979 (10.481, -21.5207) -> (10.5643, -21.5207) construction
  spline S188 degree 2 poles (10.5643, -21.5207) (10.6302, -21.5207) (10.6927, -21.5658) knots 0 0 0 1 1 1
  line L980 (10.5643, -21.5207) -> (10.6302, -21.5207) construction
  line L981 (10.6302, -21.5207) -> (10.6927, -21.5658) construction
  spline S189 degree 2 poles (10.6927, -21.5658) (10.9078, -21.7323) (11.1888, -21.7323) knots 0 0 0 1 1 1
  line L982 (10.6927, -21.5658) -> (10.9078, -21.7323) construction
  line L983 (10.9078, -21.7323) -> (11.1888, -21.7323) construction
  line L984 (11.1888, -21.7323) -> (11.3969, -21.7323)
  spline S190 degree 2 poles (11.3969, -21.7323) (11.5947, -21.7323) (11.7092, -21.6005) knots 0 0 0 1 1 1
  line L985 (11.3969, -21.7323) -> (11.5947, -21.7323) construction
  line L986 (11.5947, -21.7323) -> (11.7092, -21.6005) construction
  spline S191 degree 2 poles (11.7092, -21.6005) (11.8132, -21.4825) (11.8132, -21.3125) knots 0 0 0 1 1 1
  line L987 (11.7092, -21.6005) -> (11.8132, -21.4825) construction
  line L988 (11.8132, -21.4825) -> (11.8132, -21.3125) construction
  spline S192 degree 2 poles (11.8132, -21.3125) (11.8132, -20.9413) (11.4524, -20.9031) knots 0 0 0 1 1 1
  line L989 (11.8132, -21.3125) -> (11.8132, -20.9413) construction
  line L990 (11.8132, -20.9413) -> (11.4524, -20.9031) construction
  line L991 (11.4524, -20.9031) -> (11.1922, -20.9031)
  spline S193 degree 2 poles (-18.3883, -34.8092) (-18.5964, -34.8092) (-18.5964, -34.601) knots 0 0 0 1 1 1
  line L992 (-18.3883, -34.8092) -> (-18.5964, -34.8092) construction
  line L993 (-18.5964, -34.8092) -> (-18.5964, -34.601) construction
  line L994 (-18.5964, -34.601) -> (-18.5964, -30.8646)
  spline S194 degree 2 poles (-18.5964, -30.8646) (-18.5964, -30.6564) (-18.3883, -30.6564) knots 0 0 0 1 1 1
  line L995 (-18.5964, -30.8646) -> (-18.5964, -30.6564) construction
  line L996 (-18.5964, -30.6564) -> (-18.3883, -30.6564) construction
  spline S195 degree 2 poles (-18.3883, -30.6564) (-18.1801, -30.6564) (-18.1801, -30.8646) knots 0 0 0 1 1 1
  line L997 (-18.3883, -30.6564) -> (-18.1801, -30.6564) construction
  line L998 (-18.1801, -30.6564) -> (-18.1801, -30.8646) construction
  spline S196 degree 2 poles (-16.7265, -34.3929) (-16.5183, -34.3929) (-16.5183, -34.601) knots 0 0 0 1 1 1
  line L999 (-16.7265, -34.3929) -> (-16.5183, -34.3929) construction
  line L1000 (-16.5183, -34.3929) -> (-16.5183, -34.601) construction
  spline S197 degree 2 poles (-16.5183, -34.601) (-16.5183, -34.8092) (-16.7265, -34.8092) knots 0 0 0 1 1 1
  line L1001 (-16.5183, -34.601) -> (-16.5183, -34.8092) construction
  line L1002 (-16.5183, -34.8092) -> (-16.7265, -34.8092) construction
  line L1003 (-16.7265, -34.8092) -> (-18.3883, -34.8092)
  spline S198 degree 2 poles (-19.795, -25.6945) (-19.795, -25.7777) (-19.9199, -25.9096) (-20.0032, -25.9096) knots 0 0 0 1 2 2 2
  line L1004 (-19.795, -25.6945) -> (-19.795, -25.7777) construction
  line L1005 (-19.795, -25.7777) -> (-19.9199, -25.9096) construction
  line L1006 (-19.9199, -25.9096) -> (-20.0032, -25.9096) construction
  spline S199 degree 2 poles (-20.0032, -25.9096) (-20.0691, -25.9096) (-20.1281, -25.8679) knots 0 0 0 1 1 1
  line L1007 (-20.0032, -25.9096) -> (-20.0691, -25.9096) construction
  line L1008 (-20.0691, -25.9096) -> (-20.1281, -25.8679) construction
  spline S200 degree 2 poles (-20.1281, -25.8679) (-20.5236, -25.5834) (-21.0058, -25.5834) knots 0 0 0 1 1 1
  line L1009 (-20.1281, -25.8679) -> (-20.5236, -25.5834) construction
  line L1010 (-20.5236, -25.5834) -> (-21.0058, -25.5834) construction
  spline S201 degree 2 poles (-21.0058, -25.5834) (-21.3181, -25.5834) (-21.8211, -25.8436) (-21.8211, -26.0934) knots 0 0 0 1 2 2 2
  line L1011 (-21.0058, -25.5834) -> (-21.3181, -25.5834) construction
  line L1012 (-21.3181, -25.5834) -> (-21.8211, -25.8436) construction
  line L1013 (-21.8211, -25.8436) -> (-21.8211, -26.0934) construction
  spline S202 degree 2 poles (-21.8211, -26.0934) (-21.8211, -26.2426) (-21.7031, -26.3328) knots 0 0 0 1 1 1
  line L1014 (-21.8211, -26.0934) -> (-21.8211, -26.2426) construction
  line L1015 (-21.8211, -26.2426) -> (-21.7031, -26.3328) construction
  line L1016 (-21.7031, -26.3328) -> (-20.1628, -27.4708)
  spline S203 degree 2 poles (-20.1628, -27.4708) (-19.7464, -27.7761) (-19.7464, -28.3242) knots 0 0 0 1 1 1
  line L1017 (-20.1628, -27.4708) -> (-19.7464, -27.7761) construction
  line L1018 (-19.7464, -27.7761) -> (-19.7464, -28.3242) construction
  spline S204 degree 2 poles (-19.7464, -28.3242) (-19.7464, -28.8932) (-20.6207, -29.3511) (-21.0405, -29.3511) knots 0 0 0 1 2 2 2
  line L1019 (-19.7464, -28.3242) -> (-19.7464, -28.8932) construction
  line L1020 (-19.7464, -28.8932) -> (-20.6207, -29.3511) construction
  line L1021 (-20.6207, -29.3511) -> (-21.0405, -29.3511) construction
  spline S205 degree 2 poles (-21.0405, -29.3511) (-21.5678, -29.3511) (-22.1403, -28.9799) knots 0 0 0 1 1 1
  line L1022 (-21.0405, -29.3511) -> (-21.5678, -29.3511) construction
  line L1023 (-21.5678, -29.3511) -> (-22.1403, -28.9799) construction
  spline S206 degree 2 poles (-22.1403, -28.9799) (-22.2374, -28.9175) (-22.2374, -28.8134) knots 0 0 0 1 1 1
  line L1024 (-22.1403, -28.9799) -> (-22.2374, -28.9175) construction
  line L1025 (-22.2374, -28.9175) -> (-22.2374, -28.8134) construction
  spline S207 degree 2 poles (-22.2374, -28.8134) (-22.2374, -28.7267) (-22.116, -28.5948) (-22.0293, -28.5948) knots 0 0 0 1 2 2 2
  line L1026 (-22.2374, -28.8134) -> (-22.2374, -28.7267) construction
  line L1027 (-22.2374, -28.7267) -> (-22.116, -28.5948) construction
  line L1028 (-22.116, -28.5948) -> (-22.0293, -28.5948) construction
  spline S208 degree 2 poles (-22.0293, -28.5948) (-21.9703, -28.5948) (-21.9182, -28.633) knots 0 0 0 1 1 1
  line L1029 (-22.0293, -28.5948) -> (-21.9703, -28.5948) construction
  line L1030 (-21.9703, -28.5948) -> (-21.9182, -28.633) construction
  spline S209 degree 2 poles (-21.9182, -28.633) (-21.4464, -28.9348) (-21.0301, -28.9348) knots 0 0 0 1 1 1
  line L1031 (-21.9182, -28.633) -> (-21.4464, -28.9348) construction
  line L1032 (-21.4464, -28.9348) -> (-21.0301, -28.9348) construction
  spline S210 degree 2 poles (-21.0301, -28.9348) (-20.7109, -28.9348) (-20.3744, -28.7614) knots 0 0 0 1 1 1
  line L1033 (-21.0301, -28.9348) -> (-20.7109, -28.9348) construction
  line L1034 (-20.7109, -28.9348) -> (-20.3744, -28.7614) construction
  spline S211 degree 2 poles (-20.3744, -28.7614) (-20.1489, -28.6399) (-20.1489, -28.3312) knots 0 0 0 1 1 1
  line L1035 (-20.3744, -28.7614) -> (-20.1489, -28.6399) construction
  line L1036 (-20.1489, -28.6399) -> (-20.1489, -28.3312) construction
  spline S212 degree 2 poles (-20.1489, -28.3312) (-20.1489, -27.9946) (-20.3952, -27.8142) knots 0 0 0 1 1 1
  line L1037 (-20.1489, -28.3312) -> (-20.1489, -27.9946) construction
  line L1038 (-20.1489, -27.9946) -> (-20.3952, -27.8142) construction
  line L1039 (-20.3952, -27.8142) -> (-21.9356, -26.6728)
  spline S213 degree 2 poles (-21.9356, -26.6728) (-22.2201, -26.4647) (-22.2201, -26.0865) knots 0 0 0 1 1 1
  line L1040 (-21.9356, -26.6728) -> (-22.2201, -26.4647) construction
  line L1041 (-22.2201, -26.4647) -> (-22.2201, -26.0865) construction
  spline S214 degree 2 poles (-22.2201, -26.0865) (-22.2201, -25.5904) (-21.7587, -25.3475) knots 0 0 0 1 1 1
  line L1042 (-22.2201, -26.0865) -> (-22.2201, -25.5904) construction
  line L1043 (-22.2201, -25.5904) -> (-21.7587, -25.3475) construction
  spline S215 degree 2 poles (-21.7587, -25.3475) (-21.4256, -25.1775) (-21.0058, -25.1775) knots 0 0 0 1 1 1
  line L1044 (-21.7587, -25.3475) -> (-21.4256, -25.1775) construction
  line L1045 (-21.4256, -25.1775) -> (-21.0058, -25.1775) construction
  spline S216 degree 2 poles (-21.0058, -25.1775) (-20.3813, -25.1775) (-19.8887, -25.5279) knots 0 0 0 1 1 1
  line L1046 (-21.0058, -25.1775) -> (-20.3813, -25.1775) construction
  line L1047 (-20.3813, -25.1775) -> (-19.8887, -25.5279) construction
  spline S217 degree 2 poles (-19.8887, -25.5279) (-19.795, -25.5939) (-19.795, -25.6945) knots 0 0 0 1 1 1
  line L1048 (-19.8887, -25.5279) -> (-19.795, -25.5939) construction
  line L1049 (-19.795, -25.5939) -> (-19.795, -25.6945) construction
  spline S218 degree 2 poles (-6.2745, -21.78) (-6.0802, -21.78) (-5.9658, -21.6516) knots 0 0 0 1 1 1
  line L1050 (-6.2745, -21.78) -> (-6.0802, -21.78) construction
  line L1051 (-6.0802, -21.78) -> (-5.9658, -21.6516) construction
  spline S219 degree 2 poles (-5.9658, -21.6516) (-5.8617, -21.5337) (-5.8617, -21.3637) knots 0 0 0 1 1 1
  line L1052 (-5.9658, -21.6516) -> (-5.8617, -21.5337) construction
  line L1053 (-5.8617, -21.5337) -> (-5.8617, -21.3637) construction
  spline S220 degree 2 poles (-5.8617, -21.3637) (-5.8617, -21.1937) (-5.9658, -21.0792) knots 0 0 0 1 1 1
  line L1054 (-5.8617, -21.3637) -> (-5.8617, -21.1937) construction
  line L1055 (-5.8617, -21.1937) -> (-5.9658, -21.0792) construction
  spline S221 degree 2 poles (-5.9658, -21.0792) (-6.0802, -20.9508) (-6.2745, -20.9508) knots 0 0 0 1 1 1
  line L1056 (-5.9658, -21.0792) -> (-6.0802, -20.9508) construction
  line L1057 (-6.0802, -20.9508) -> (-6.2745, -20.9508) construction
  spline S222 degree 2 poles (-6.2745, -20.5345) (-5.879, -20.5345) (-5.6535, -20.7947) knots 0 0 0 1 1 1
  line L1058 (-6.2745, -20.5345) -> (-5.879, -20.5345) construction
  line L1059 (-5.879, -20.5345) -> (-5.6535, -20.7947) construction
  spline S223 degree 2 poles (-5.6535, -20.7947) (-5.4454, -21.0272) (-5.4454, -21.3637) knots 0 0 0 1 1 1
  line L1060 (-5.6535, -20.7947) -> (-5.4454, -21.0272) construction
  line L1061 (-5.4454, -21.0272) -> (-5.4454, -21.3637) construction
  spline S224 degree 2 poles (-5.4454, -21.3637) (-5.4454, -21.7002) (-5.6535, -21.9396) knots 0 0 0 1 1 1
  line L1062 (-5.4454, -21.3637) -> (-5.4454, -21.7002) construction
  line L1063 (-5.4454, -21.7002) -> (-5.6535, -21.9396) construction
  spline S225 degree 2 poles (-5.6535, -21.9396) (-5.8825, -22.1963) (-6.2745, -22.1963) knots 0 0 0 1 1 1
  line L1064 (-5.6535, -21.9396) -> (-5.8825, -22.1963) construction
  line L1065 (-5.8825, -22.1963) -> (-6.2745, -22.1963) construction
  line L1066 (-6.2745, -22.1963) -> (-7.3119, -22.1963)
  spline S226 degree 2 poles (-7.3119, -22.1963) (-7.52, -22.1963) (-7.52, -21.9882) knots 0 0 0 1 1 1
  line L1067 (-7.3119, -22.1963) -> (-7.52, -22.1963) construction
  line L1068 (-7.52, -22.1963) -> (-7.52, -21.9882) construction
  line L1069 (-7.52, -21.9882) -> (-7.52, -19.4972)
  spline S227 degree 2 poles (-7.52, -19.4972) (-7.52, -19.289) (-7.3119, -19.289) knots 0 0 0 1 1 1
  line L1070 (-7.52, -19.4972) -> (-7.52, -19.289) construction
  line L1071 (-7.52, -19.289) -> (-7.3119, -19.289) construction
  spline S228 degree 2 poles (-7.3119, -19.289) (-7.1037, -19.289) (-7.1037, -19.4972) knots 0 0 0 1 1 1
  line L1072 (-7.3119, -19.289) -> (-7.1037, -19.289) construction
  line L1073 (-7.1037, -19.289) -> (-7.1037, -19.4972) construction
  line L1074 (-11.0518, -22.1963) -> (-12.0891, -22.1963)
  spline S229 degree 2 poles (-12.0891, -22.1963) (-12.4291, -22.1963) (-12.9183, -21.7106) (-12.9183, -21.3672) knots 0 0 0 1 2 2 2
  line L1075 (-12.0891, -22.1963) -> (-12.4291, -22.1963) construction
  line L1076 (-12.4291, -22.1963) -> (-12.9183, -21.7106) construction
  line L1077 (-12.9183, -21.7106) -> (-12.9183, -21.3672) construction
  line L1078 (-12.9183, -21.3672) -> (-12.9183, -19.4972)
  spline S230 degree 2 poles (-12.9183, -19.4972) (-12.9183, -19.289) (-12.7101, -19.289) knots 0 0 0 1 1 1
  line L1079 (-12.9183, -19.4972) -> (-12.9183, -19.289) construction
  line L1080 (-12.9183, -19.289) -> (-12.7101, -19.289) construction
  spline S231 degree 2 poles (-12.7101, -19.289) (-12.502, -19.289) (-12.502, -19.4972) knots 0 0 0 1 1 1
  line L1081 (-12.7101, -19.289) -> (-12.502, -19.289) construction
  line L1082 (-12.502, -19.289) -> (-12.502, -19.4972) construction
  line L1083 (-12.502, -19.4972) -> (-12.502, -21.3637)
  spline S232 degree 2 poles (-12.502, -21.3637) (-12.502, -21.5337) (-12.2591, -21.78) (-12.0891, -21.78) knots 0 0 0 1 2 2 2
  line L1084 (-12.502, -21.3637) -> (-12.502, -21.5337) construction
  line L1085 (-12.502, -21.5337) -> (-12.2591, -21.78) construction
  line L1086 (-12.2591, -21.78) -> (-12.0891, -21.78) construction
  spline S233 degree 2 poles (-11.26, -19.4972) (-11.26, -19.289) (-11.0518, -19.289) knots 0 0 0 1 1 1
  line L1087 (-11.26, -19.4972) -> (-11.26, -19.289) construction
  line L1088 (-11.26, -19.289) -> (-11.0518, -19.289) construction
  spline S234 degree 2 poles (-11.0518, -19.289) (-10.8436, -19.289) (-10.8436, -19.4972) knots 0 0 0 1 1 1
  line L1089 (-11.0518, -19.289) -> (-10.8436, -19.289) construction
  line L1090 (-10.8436, -19.289) -> (-10.8436, -19.4972) construction
  line L1091 (-10.8436, -19.4972) -> (-10.8436, -21.9882)
  spline S235 degree 2 poles (-10.8436, -21.9882) (-10.8436, -22.1963) (-11.0518, -22.1963) knots 0 0 0 1 1 1
  line L1092 (-10.8436, -21.9882) -> (-10.8436, -22.1963) construction
  line L1093 (-10.8436, -22.1963) -> (-11.0518, -22.1963) construction
  spline S236 degree 2 poles (-20.6029, -20.9508) (-20.811, -20.9508) (-20.811, -20.7427) knots 0 0 0 1 1 1
  line L1094 (-20.6029, -20.9508) -> (-20.811, -20.9508) construction
  line L1095 (-20.811, -20.9508) -> (-20.811, -20.7427) construction
  spline S237 degree 2 poles (-20.811, -20.7427) (-20.811, -20.5345) (-20.6029, -20.5345) knots 0 0 0 1 1 1